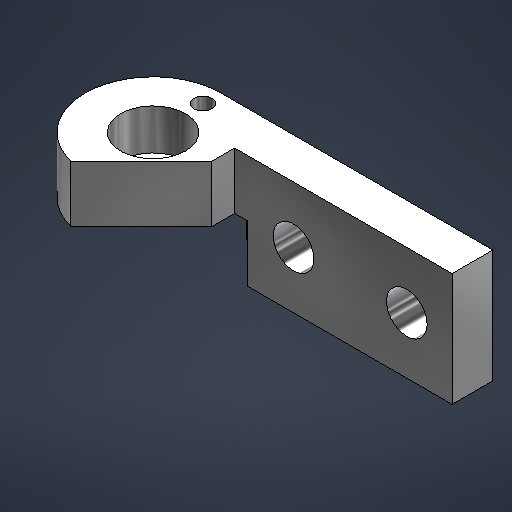
# Autodesk Inventor part: 2DU81
Saved by Autodesk Inventor 2026.1 (Build 301233020, 233B)
## iProperties
Manager: 100-52946
Category: _
Created: 2013-06-10
Material: Aluminum 6061
Document SubType Name: Modeling
Designer: caitlin.parks , Caitlin
Manufacturer: Standard
Standards Organization: Custom
Checked By: 2DU81
Engr Approved By: P
User Status: Released
Description: BRACKET, ADJUSTABLE ANGLE, KEYED, MK40MM
Mass: 41.0664 g
Surface Area: 66.6645 cm^2
Volume: 15.2098 cm^3
Density: 2.7 g/cm^3
Mfg Approved By: Stephen.Oerton
Appearance: Aluminum - Flat
Part Number: 2DU81
CN_SERVICEABLE: _
CN_MASS: 0.38706572297471525
CL_runCount: 1
FIRST_DESCRIPTION: _
SECOND_DESCRIPTION: _
THIRD_DESCRIPTION: _
Author: -
Subject: B46.00.020
Keywords: MK
Revision Number: 1
Autodesk Inventor part; units mm, degrees
ref_plane "YZ Plane" through (0, 0, 0) normal (1, 0, 0) x (0, 1, 0)
ref_plane "XZ Plane" through (0, 0, 0) normal (0, 1, 0) x (-1, 0, 0)
ref_plane "XY Plane" through (0, 0, 0) normal (0, 0, 1) x (1, 0, 0)
sketch "Sketch2" plane through (0, 0, 0) normal (0, 1, 0) x (-1, 0, 0)
  line L0 (-60, -6) -> (-60, -15)
  line L1 (-60, -15) -> (0, -15)
  arc A0 (0, -15) -> (3.5692, 14.5692) centre (0, 0) ccw
  line L2 (3.5692, 14.5692) -> (-12, -1)
  line L3 (-12, -1) -> (-12, -6)
  line L4 (-12, -6) -> (-60, -6)
  dimension "d1" = 15
  dimension "d2" = 60
  dimension "d3" = 9
  dimension "d4" = 45
  dimension "d5" = 5
  dimension "d6" = 7.7782
  constraints: 10 end point, 2 perpendicular, 2 point on circle, 2 vertical, 1 centre point, 1 coincident, 1 tangent
  measures "d1" radius of A0
  measures "d2" distance of L0.end L1.end
  measures "d3" distance of L0.start L0.end
  measures "d4" angle of L2 L4
  measures "d5" distance of L2.end L3.end
  measures "d6" distance from line of point (0, 0) L2
extrude "Extrusion1" add sketch "Sketch2" along normal mid plane 25
sketch "Sketch3" plane through (0, -12.5, 0) normal (0, -1, 0) x (1, 0, 0)
  point P0 (0, 0)
  point P1 (0, 0)
  constraints: 1 coincident
hole "Hole1" at (0, -12.5, 0) direction (0, 1, 0) diameter 32 depth 12.5
sketch "Sketch4" plane through (0, 12.5, 0) normal (0, 1, 0) x (1, 0, 0)
  point P0 (0, 0)
  point P1 (0, 0)
  constraints: 1 coincident
hole "Hole2" at (0, 12.5, 0) direction (0, -1, 0) diameter 9 end through all counterbore diameter 14.3 counterbore depth 9
sketch "Sketch5" plane through (0, 12.5, 0) normal (0, 1, 0) x (1, 0, 0)
  line L0 (0, 0) -> (0, 11) construction
  dimension "d23" = 11
  constraints: 2 end point, 1 vertical
  measures "d23" distance of L0.start L0.end
hole "Hole3" at (0, 12.5, -11) direction (0, -1, 0) diameter 4 end through all
sketch "Sketch6" plane through (12, 12.5, -6) normal (0, 0, 1) x (1, 0, 0)
  line L0 (-42, -12.5) -> (63, -12.5) construction
  line L1 (48, -25) -> (48, 0) construction
  point P0 (-12, -12.5)
  point P1 (38, -12.5)
  point P2 (13, -12.5)
  dimension "d31" = 25
  dimension "d32" = 10
  constraints: 2 point on line
  measures "d31" distance of point (13, -12.5) point (38, -12.5)
  measures "d32" distance from line of L1 point (38, -12.5)
hole "Hole4" at (50, 0, -6) at (25, 0, -6) direction (0, 0, -1) diameter 9 end through all
equation "\"d14\" = 0.5 * d7"
equation "\"d21\" = 0.5 * d7"
equation "\"d7\" = 25"
